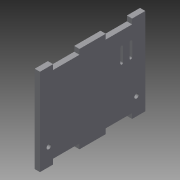
# Autodesk Inventor part: SideLeft
Saved by Autodesk Inventor 2015 (Build 190159000, 159)
## iProperties
Created: 2017-03-04
Part Number: SideLeft
Material: Generic
Document SubType Name: Modeling
Designer: Guy
Density: 1 g/cm^3
Appearance: Default
Author: Guy
Autodesk Inventor part; units mm, degrees
ref_plane "YZ Plane" through (0, 0, 0) normal (1, 0, 0) x (0, 1, 0)
ref_plane "XZ Plane" through (0, 0, 0) normal (0, 1, 0) x (-1, 0, 0)
ref_plane "XY Plane" through (0, 0, 0) normal (0, 0, 1) x (1, 0, 0)
sketch "Sketch1" plane through (0, 0, 0) normal (1, 0, 0) x (0, 1, 0)
  line L0 (0, 0) -> (120, 0)
  line L1 (120, 0) -> (120, -99)
  line L2 (120, -99) -> (0, -99)
  line L3 (0, -99) -> (0, 0)
  dimension "d0" = 120
  dimension "d1" = 99
  constraints: 8 end point, 2 parallel, 1 horizontal, 1 perpendicular
  measures "d0" distance of L1.end L2.end
  measures "d1" distance of L0.end L1.end
extrude "Extrusion1" add sketch "Sketch1" along normal blind 6
sketch "Sketch2" plane through (6, 0, 0) normal (1, 0, 0) x (0, 0, -1)
  line L0 (0, 120) -> (0, 0) projected
  line L1 (0, 0) -> (99, 0) projected
  line L2 (99, 0) -> (99, 120) projected
  line L3 (99, 120) -> (0, 120) projected
  line L4 (0, 120) -> (0, 0) projected
  line L5 (0, 15) -> (5.75, 15)
  line L6 (5.75, 15) -> (5.75, 45)
  line L7 (5.75, 45) -> (0, 45)
  line L8 (0, 45) -> (0, 15)
  line L9 (0, 75) -> (5.75, 75)
  line L10 (5.75, 75) -> (5.75, 105)
  line L11 (5.75, 105) -> (0, 105)
  line L12 (0, 105) -> (0, 75)
  line L13 (99, 15) -> (93.25, 15)
  line L14 (93.25, 15) -> (93.25, 45)
  line L15 (93.25, 45) -> (99, 45)
  line L16 (99, 45) -> (99, 15)
  line L17 (99, 75) -> (93.25, 75)
  line L18 (93.25, 75) -> (93.25, 105)
  line L19 (93.25, 105) -> (99, 105)
  line L20 (99, 105) -> (99, 75)
  line L21 (-12.0657, 60) -> (104.2665, 60)
  line L22 (99, 120) -> (0, 120) projected
  dimension "d5" = 5.75
  dimension "d6" = 5.75
  dimension "d8" = 30
  dimension "d9" = 30
  dimension "d22" = 60
  dimension "d23" = 15
  dimension "d24" = 15
  constraints: 34 end point, 9 parallel, 5 collinear, 5 horizontal, 5 point on line, 4 perpendicular
  measures "d5" distance between parallel lines of L10 L0
  measures "d6" distance between parallel lines of L20 L18
  measures "d8" distance between parallel lines of L19 L17
  measures "d9" distance between parallel lines of L13 L15
  measures "d22" distance between parallel lines of L21 L3
  measures "d23" distance between parallel lines of L17 L21
  measures "d24" distance between parallel lines of L15 L21
extrude "Extrusion2" cut sketch "Sketch2" against normal up to next contours L11 L10 L9 L0 | L2 L17 L18 L19 | L7 L6 L5 L0 | L2 L13 L14 L15
sketch "Sketch3" plane through (6, 0, 0) normal (1, 0, 0) x (0, 0, -1)
  circle A0 centre (79, 10) radius 2.5
  circle A1 centre (79, 110) radius 2.5
  line L0 (99, 105) -> (99, 120) projected
  line L1 (99, 120) -> (0, 120) projected
  line L2 (99, 0) -> (99, 15) projected
  line L3 (0, 0) -> (99, 0) projected
  dimension "d13" = 20
  dimension "d14" = 10
  dimension "d15" = 5
  dimension "d17" = 10
  dimension "d18" = 20
  dimension "d19" = 5
  constraints: 2 centre point
  measures "d13" distance from line of L0 A1.centre
  measures "d14" distance from line of A1.centre L1
  measures "d15" diameter of A1
  measures "d17" distance from line of A0.centre L3
  measures "d18" distance from line of A0.centre L2
  measures "d19" diameter of A0
extrude "Extrusion3" cut sketch "Sketch3" against normal up to next
sketch "Sketch4" plane through (6, 0, 0) normal (1, 0, 0) x (0, 0, -1)
  circle A0 centre (79, 10) radius 2.5 projected
  circle A1 centre (79, 110) radius 2.5 projected
  line L0 (5.75, 75) -> (0, 75) projected
  line L1 (0, 75) -> (0, 45) projected
  line L2 (0, 45) -> (5.75, 45) projected
  line L3 (5.75, 45) -> (5.75, 15) projected
  line L4 (5.75, 15) -> (0, 15) projected
  line L5 (0, 15) -> (0, 0) projected
  line L6 (0, 0) -> (99, 0) projected
  line L7 (99, 0) -> (99, 15) projected
  line L8 (99, 15) -> (93.25, 15) projected
  line L9 (93.25, 15) -> (93.25, 45) projected
  line L10 (93.25, 45) -> (99, 45) projected
  line L11 (99, 45) -> (99, 75) projected
  line L12 (99, 75) -> (93.25, 75) projected
  line L13 (93.25, 75) -> (93.25, 105) projected
  line L14 (93.25, 105) -> (99, 105) projected
  line L15 (99, 105) -> (99, 120) projected
  line L16 (99, 120) -> (0, 120) projected
  line L17 (0, 120) -> (0, 105) projected
  line L18 (0, 105) -> (5.75, 105) projected
  line L19 (5.75, 105) -> (5.75, 75) projected
  circle A2 centre (33.095, 103.598) radius 1.5 construction
  circle A3 centre (33.095, 93.242) radius 1.5 construction
  arc A4 (22.095, 105.098) -> (22.095, 102.098) centre (22.095, 103.598) ccw
  arc A5 (38.095, 102.098) -> (38.095, 105.098) centre (38.095, 103.598) ccw
  arc A6 (22.095, 94.742) -> (22.095, 91.742) centre (22.095, 93.242) ccw
  arc A7 (38.095, 91.742) -> (38.095, 94.742) centre (38.095, 93.242) ccw
  line L20 (22.095, 91.742) -> (38.095, 91.742)
  line L21 (22.095, 94.742) -> (38.095, 94.742)
  line L22 (22.095, 102.098) -> (38.095, 102.098)
  line L23 (22.095, 105.098) -> (38.095, 105.098)
  dimension "d25" = 3
  dimension "d26" = 3
  dimension "d27" = 10.356
  dimension "d28" = 16.402
  dimension "d29" = 65.905
  dimension "d30" = 3
  dimension "d31" = 3
  dimension "d32" = 3
  dimension "d33" = 3
  dimension "d34" = 16
  dimension "d35" = 16
  dimension "d36" = 11
  dimension "d37" = 11
  constraints: 8 end point, 8 point on circle, 8 tangent, 6 centre point
  measures "d25" diameter of A2
  measures "d26" diameter of A3
  measures "d27" distance of A3.centre A2.centre
  measures "d28" distance from line of L16 A2.centre
  measures "d29" distance from line of L15 A2.centre
  measures "d30" diameter of A6
  measures "d31" diameter of A4
  measures "d32" diameter of A5
  measures "d33" diameter of A7
  measures "d34" distance of A7.centre A6.centre
  measures "d35" distance of A5.centre A4.centre
  measures "d36" distance of A2.centre A4.centre
  measures "d37" distance of A3.centre A6.centre
extrude "Extrusion4" cut sketch "Sketch4" against normal blind 10 contours L23 A5 L22 A4 | L21 A7 L20 A6
equation "\"d26\" = d25"
equation "\"d30\" = d25"
equation "\"d31\" = d25"
equation "\"d32\" = d25"
equation "\"d33\" = d25"
body "Solid1"
